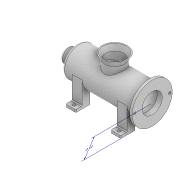
# Autodesk Inventor part: Carcasa
Saved by Autodesk Inventor 2021 (Build 250183000, 183)
## iProperties
Created: 2022-02-09
Part Number: Carcasa
Material: Aluminum
Document SubType Name: Modeling
Designer: Santiago
Density: 2.7 g/cm^3
Appearance: Aluminum Cast
Author: Santiago
Autodesk Inventor part; units mm, degrees
ref_plane "YZ Plane" through (0, 0, 0) normal (1, 0, 0) x (0, 1, 0)
ref_plane "XY Plane" through (0, 0, 0) normal (0, 0, 1) x (1, 0, 0)
sketch "Sketch1" plane through (0, 0, 0) normal (0, 0, 1) x (1, 0, 0)
  line L0 (0, 0) -> (-130.3125, 0)
  line L1 (-130.3125, 0) -> (-130.3125, 9.2875)
  line L2 (-125.3125, 14.2875) -> (-112.3125, 14.2875)
  line L3 (-110.3125, 16.2875) -> (-110.3125, 25)
  line L4 (-105.3125, 30) -> (34.6875, 30)
  line L5 (39.6875, 25) -> (39.6875, 0)
  line L6 (39.6875, 0) -> (-130.3125, 0)
  arc A0 (-112.3125, 14.2875) -> (-110.3125, 16.2875) centre (-112.3125, 16.2875) ccw
  arc A1 (-105.3125, 30) -> (-110.3125, 25) centre (-105.3125, 25) ccw
  arc A2 (-125.3125, 14.2875) -> (-130.3125, 9.2875) centre (-125.3125, 9.2875) ccw
  arc A3 (39.6875, 25) -> (34.6875, 30) centre (34.6875, 25) ccw
  point P0 (-130.3125, 14.2875)
  point P1 (-110.3125, 14.2875)
  point P2 (-110.3125, 30)
  point P3 (39.6875, 30)
  dimension "d7" = 14.2875
  dimension "d8" = 150
  dimension "d9" = 20
  dimension "d10" = 30
  dimension "d17" = 2
  dimension "d18" = 5
  dimension "d19" = 5
  constraints: 14 end point, 9 point on line, 8 point on circle, 8 tangent, 6 perpendicular, 4 centre point, 1 equal radius, 1 horizontal
  measures "d7" distance of L0.end point (-130.312, 14.288)
  measures "d8" distance of point (-110.312, 30) point (39.688, 30)
  measures "d9" distance of point (-130.312, 14.288) point (-110.312, 14.287)
  measures "d10" distance of point (39.688, 30) L5.end
  measures "d17" radius of A0
  measures "d18" radius of A1
  measures "d19" radius of A2
revolve "Revolution1" add sketch "Sketch1" angle 360 about axis through (39.6875, 0, 0) along (-1, 0, 0)
sketch "Sketch3" plane through (39.6875, 0, 0) normal (1, 0, 0) x (0, 0, -1)
  circle A0 centre (0, 0) radius 27.5
  dimension "d11" = 55
  constraints: 1 centre point, 1 coincident
  measures "d11" diameter of A0
extrude "Extrusion2" cut sketch "Sketch3" against normal blind 145
sketch "Sketch4" plane through (-130.3125, 0, 0) normal (-1, 0, 0) x (0, 0, 1)
  circle A0 centre (0, 0) radius 7.5
  dimension "d14" = 15
  constraints: 1 centre point, 1 coincident
  measures "d14" diameter of A0
extrude "Extrusion3" cut sketch "Sketch4" against normal through all
ref_plane "Work Plane1" through (-35.3125, 30, 0) normal (0, 1, 0) x (-1, 0, 0)
sketch "Sketch5" plane through (-35.3125, 30, 0) normal (0, 1, 0) x (-1, 0, 0)
  circle A0 centre (0, 0) radius 20
  circle A1 centre (0, 0) radius 18
  point P0 (-35.3125, 0)
  dimension "d20" = 40
  dimension "d21" = 36
  constraints: 2 centre point, 1 coincident
  measures "d20" diameter of A0
  measures "d21" diameter of A1
extrude "Extrusion4" add sketch "Sketch5" against normal up to next
extrude "Extrusion5" add sketch "Sketch5" along normal blind 10
extrude "Extrusion6" cut sketch "Sketch5" against normal blind 10 contours A1
ref_plane "Work Plane3" through (-35.3125, 50, 0) normal (0, 1, 0) x (1, 0, 0)
ref_plane "Work Plane2" through (-35.3125, 40, 0) normal (0, 1, 0) x (1, 0, 0)
sketch "Sketch6" plane through (-35.3125, 50, 0) normal (0, 1, 0) x (1, 0, 0)
  circle A0 centre (0, 0) radius 25
  circle A1 centre (0, 0) radius 23
  point P0 (35.3125, 0)
  dimension "d30" = 50
  dimension "d31" = 46
  constraints: 2 centre point, 1 coincident
  measures "d30" diameter of A0
  measures "d31" diameter of A1
loft "Loft1" add profiles "Sketch6" section 1 edges at (-15.3125, 40, 0) contours A0 | A1
sketch "Sketch7" plane through (-35.3125, 50, 0) normal (0, 1, 0) x (1, 0, 0)
  circle A0 centre (0, 0) radius 23
  point P0 (35.3125, 0)
  dimension "d36" = 46
  constraints: 1 centre point
  measures "d36" diameter of A0
sketch "Sketch9" plane through (-35.3125, 40, 0) normal (0, 1, 0) x (1, 0, 0)
  circle A0 centre (0, 0) radius 18
  point P0 (35.3125, 0)
  dimension "d37" = 36
  constraints: 1 centre point
  measures "d37" diameter of A0
loft "Loft2" cut profiles "Sketch7" section 2 edges at (-17.3125, 40, 0)
ref_plane "Work Plane4" through (39.6875, 0, 0) normal (-1, 0, 0) x (0, 0, 1)
sketch "Sketch10" plane through (39.6875, 0, 0) normal (-1, 0, 0) x (0, 0, 1)
  circle A0 centre (0, 0) radius 27.5
  circle A1 centre (0, 0) radius 40
  dimension "d43" = 80
  constraints: 2 centre point, 2 coincident
  measures "d43" diameter of A1
extrude "Extrusion7" add sketch "Sketch10" along normal blind 5
sketch "Sketch11" plane through (39.6875, 0, 0) normal (-1, 0, 0) x (0, 0, 1)
  circle A0 centre (35, 0) radius 2.5
  line L0 (-18, 40) -> (18, 40) projected
  line L1 (0, 40) -> (0, -40)
  circle A1 centre (0, 0) radius 40 projected
  circle A2 centre (-35, 0) radius 2.5
  dimension "d46" = 5
  constraints: 2 centre point, 2 end point, 1 midpoint, 1 point on circle, 1 symmetric about line, 1 vertical, 1 other
  measures "d46" diameter of A0
extrude "Extrusion8" cut sketch "Sketch11" along normal blind 10 contours A0 | A2
sketch "Sketch12" plane through (39.6875, 0, 0) normal (-1, 0, 0) x (0, 0, 1)
  circle A0 centre (0, 0) radius 20
  circle A1 centre (0, 0) radius 27.5
  dimension "d49" = 40
  constraints: 2 centre point, 2 coincident
  measures "d49" diameter of A0
extrude "Extrusion9" add sketch "Sketch12" along normal blind 10
ref_plane "Work Plane5" through (-35.3125, -30, 0) normal (0, 1, 0) x (-1, 0, 0)
sketch "Sketch13" plane through (-35.3125, -30, 0) normal (0, 1, 0) x (-1, 0, 0)
  line L0 (45, 22.5) -> (-45, 22.5)
  line L1 (-45, 22.5) -> (-45, -22.5)
  line L2 (-45, -22.5) -> (45, -22.5)
  line L3 (45, -22.5) -> (45, 22.5)
  line L4 (45, 22.5) -> (-45, -22.5) construction
  line L5 (-45, 22.5) -> (45, -22.5) construction
  line L6 (-70, -30) -> (70, -30) projected
  line L7 (-55, -15) -> (-35, -15)
  line L8 (-35, -15) -> (-35, -30)
  line L9 (-35, -30) -> (-55, -30)
  line L10 (-55, -30) -> (-55, -15)
  line L11 (-55, -15) -> (-35, -30) construction
  line L12 (-35, -15) -> (-55, -30) construction
  line L13 (0, -30) -> (0, 0)
  line L14 (0, 0) -> (-70, 0)
  line L15 (-70, -30) -> (-70, 30) projected
  line L16 (55, -15) -> (35, -15)
  line L17 (35, -15) -> (35, -30)
  line L18 (35, -30) -> (55, -30)
  line L19 (55, -30) -> (55, -15)
  line L20 (55, -15) -> (35, -30) construction
  line L21 (35, -15) -> (55, -30) construction
  line L22 (-55, 15) -> (-35, 15)
  line L23 (-35, 15) -> (-35, 30)
  line L24 (-35, 30) -> (-55, 30)
  line L25 (-55, 30) -> (-55, 15)
  line L26 (-55, 15) -> (-35, 30) construction
  line L27 (-35, 15) -> (-55, 30) construction
  line L28 (35, 15) -> (35, 30)
  line L29 (55, 15) -> (35, 15)
  line L30 (35, 30) -> (55, 30)
  line L31 (55, 15) -> (35, 30) construction
  line L32 (35, 15) -> (55, 30) construction
  line L33 (55, 30) -> (55, 15)
  point P0 (-35.3125, 0)
  point P1 (-35, -22.5)
  point P2 (-45, -15)
  dimension "d52" = 90
  dimension "d53" = 45
  dimension "d54" = 20
  constraints: 64 end point, 12 midpoint, 12 symmetric about line, 4 parallel, 2 horizontal, 2 perpendicular, 1 point on line, 1 vertical
  measures "d52" distance of L2.end L1.end
  measures "d53" distance of L1.end L0.end
  measures "d54" distance of L8.end L9.end
extrude "Extrusion10" add sketch "Sketch13" along normal up to next contours L3 L29 L28 L0 | L0 L28 L30 L33 L29 L3 | L23 L22 L1 L0 | L0 L1 L22 L25 L24 L23 | L16 L19 L6 L17 L2 L3 | L3 L2 L17 L16 | L7 L8 L2 L1 | L1 L2 L8 L6 L10 L7
extrude "Extrusion11" add sketch "Sketch13" against normal blind 20 contours L3 L29 L28 L0 | L0 L28 L30 L33 L29 L3 | L23 L22 L1 L0 | L0 L1 L22 L25 L24 L23 | L16 L19 L6 L17 L2 L3 | L3 L2 L17 L16 | L7 L8 L2 L1 | L1 L2 L8 L6 L10 L7
ref_plane "Work Plane6" through (9.6875, -50, 30) normal (0, -1, 0) x (1, 0, 0)
sketch "Sketch14" plane through (9.6875, -50, 30) normal (0, -1, 0) x (1, 0, 0)
  line L0 (-80, 0) -> (-100, 0) projected
  line L1 (-100, 0) -> (-100, -15) projected
  line L2 (-100, -15) -> (-80, -15) projected
  line L3 (-80, -15) -> (-80, 0) projected
  line L4 (-10, -15) -> (10, -15) projected
  line L5 (10, -15) -> (10, 0) projected
  line L6 (10, 0) -> (-10, 0) projected
  line L7 (-10, 0) -> (-10, -15) projected
  line L8 (-10, -60) -> (10, -60) projected
  line L9 (10, -60) -> (10, -45) projected
  line L10 (10, -45) -> (-10, -45) projected
  line L11 (-10, -45) -> (-10, -60) projected
  line L12 (-80, -60) -> (-80, -45) projected
  line L13 (-80, -45) -> (-100, -45) projected
  line L14 (-100, -45) -> (-100, -60) projected
  line L15 (-100, -60) -> (-80, -60) projected
  line L16 (-100, 0) -> (-80, 0)
  line L17 (-80, 0) -> (-80, 12.7)
  line L18 (-80, 12.7) -> (-100, 12.7)
  line L19 (-100, 12.7) -> (-100, 0)
  line L20 (25, -60) -> (-115, -60) projected
  line L21 (-45, -60) -> (-45, 15.875)
  line L22 (-10, 0) -> (10, 0)
  line L23 (10, 0) -> (-10, 0)
  line L24 (-10, 0) -> (-10, 12.7)
  line L25 (-10, 12.7) -> (10, 12.7)
  line L26 (10, 12.7) -> (10, 0)
  line L27 (6.35, -30) -> (-115, -30)
  line L28 (-115, -22.5) -> (-115, -37.5) projected
  line L29 (-80, -60) -> (-100, -60)
  line L30 (10, -60) -> (-10, -60)
  line L31 (-100, -60) -> (-80, -60)
  line L32 (-80, -60) -> (-80, -72.7)
  line L33 (-80, -72.7) -> (-100, -72.7)
  line L34 (-100, -72.7) -> (-100, -60)
  line L35 (10, -60) -> (-10, -60)
  line L36 (10, -72.7) -> (10, -60)
  line L37 (-10, -60) -> (-10, -72.7)
  line L38 (-10, -72.7) -> (10, -72.7)
  line L39 (-10, -60) -> (10, -60)
  circle A0 centre (-90, -66.35) radius 3
  circle A1 centre (0, -66.35) radius 3
  circle A2 centre (-90, 6.35) radius 3
  circle A3 centre (0, 6.35) radius 3
  point P0 (-9.6875, -30)
  point P1 (-45, -75.875)
  dimension "d62" = 6
  dimension "d63" = 6
  dimension "d64" = 6
  dimension "d65" = 6
  constraints: 44 end point, 14 symmetric about line, 4 centre point, 2 midpoint, 2 parallel, 1 horizontal, 1 perpendicular, 1 vertical
  measures "d62" diameter of A0
  measures "d63" diameter of A1
  measures "d64" diameter of A2
  measures "d65" diameter of A3
extrude "Extrusion12" add sketch "Sketch14" against normal blind 5 contours L0 L19 L18 L17 | L24 L25 L26 L6 | L8 L36 L38 L37 | L32 L33 L34 L15 | A0 | A1 | A2 | A3
fillet "Fillet1" radius 2 12 edges at (19.6875, -47.5, 42.7) (-0.3125, -47.5, 42.7) (9.6875, -45, 30) (-80.3125, -45, 30) (-70.3125, -47.5, 42.7) (-90.3125, -47.5, 42.7) (19.6875, -47.5, -42.7) (-0.3125, -47.5, -42.7) (9.6875, -45, -30) (-70.3125, -47.5, -42.7) (-90.3125, -47.5, -42.7) (-80.3125, -45, -30)
extrude "Extrusion13" cut sketch "Sketch14" against normal blind 5 contours A0 | A1 | A2 | A3
body "Solid1"
